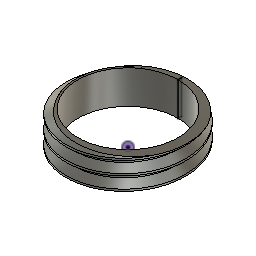
For 29mm M36x4 - 10mm high - 15mm Radius v1 (Autodesk Fusion 360 design; units mm, degrees)
Autodesk Fusion 360 part; units mm, degrees
note: some values were not read from the file. Chosen so that the rebuilt part matches the saved one: that a step has no effect. Set by a fixed rule: which sketch regions a step uses.
sketch "Sketch1" plane through (0, 0, 0) normal (1, 0, 0) x (0, 1, 0)
  line L0 (15, 0) -> (15, 10)
  line L1 (16, 10) -> (16, 0)
  line L2 (16, 0) -> (15, 0)
  line L3 (15, 10) -> (16, 10)
  dimension "d1" = 1
  dimension "d2" = 10
  dimension "d4" = 10
  dimension "d5" = 15
  constraint horizontal L2
  constraint coincident origin L2
  constraint vertical L0
  constraint vertical L1
  measures "d1" distance of L0.start L1.end
  measures "d2" distance of L0.start L0.end
  measures "d4" distance of L1.start L1.end
  measures "d5" distance of origin L0.start
revolve "Revolve1" add sketch "Sketch1" angle 360 about axis through (0, 0, 1.75) along (0, 0, 1)
thread "Thread1" "ANSI Metric M Profile 36.0 M36x4 6g" major diameter 35.7025 minor diameter 31.132 pitch 4 angle 60 modelled right hand crest width 0.5725 on face at (0.7975, 15.9801, 6.6667) crest through (0, 17.8513, -1)
extrude "Extrude4" [no effect]
